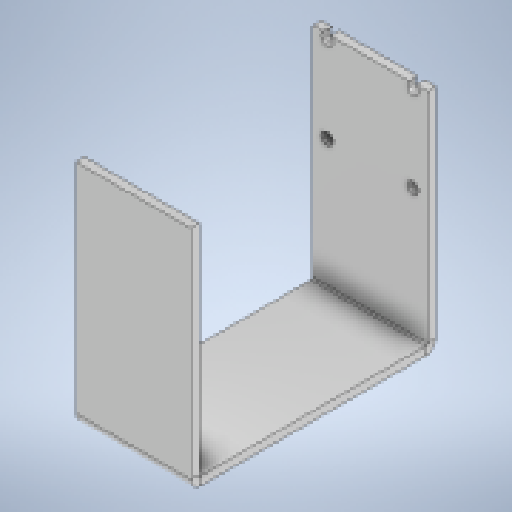
# Autodesk Inventor part: axis_25_top_frame
Saved by Autodesk Inventor 2025.2 (Build 292293000, 293)
## iProperties
Created: 2025-06-30
Part Number: axis_25_top_frame
Material: Aluminum 6061-AHC
Document SubType Name: Sheet Metal
Designer: LG
Density: 2.7 g/cm^3
Sheet Metal Rule: Default_mm
Appearance: Aluminum - Dark
Author: LG
Autodesk Inventor part; units mm, degrees
ref_plane "YZ Plane" through (0, 0, 0) normal (1, 0, 0) x (0, 1, 0)
ref_plane "XZ Plane" through (0, 0, 0) normal (0, 1, 0) x (-1, 0, 0)
ref_plane "XY Plane" through (0, 0, 0) normal (0, 0, 1) x (1, 0, 0)
sketch "Sketch1" plane through (0, 0, 0) normal (0, 1, 0) x (-1, 0, 0)
  line L0 (10.07, 20.05) -> (-10.07, 20.05)
  line L1 (-10.07, 20.05) -> (-10.07, -20.05)
  line L2 (-10.07, -20.05) -> (10.07, -20.05)
  line L3 (10.07, -20.05) -> (10.07, 20.05)
  point P0 (0, 0)
  dimension "d0" = 40.1
  dimension "d1" = 20.14
  dimension "d2" = 10.07
  dimension "d3" = 20.05
  measures "d0" distance of L2.end L0.start
  measures "d1" distance of L1.end L2.end
  measures "d2" distance from line of point (0, 0) L3
  measures "d3" distance from line of point (0, 0) L2
extrude "Plate1" add sketch "Sketch1" along normal blind 1.5
sketch "Sketch2" plane through (10.07, 0, 21.55) normal (0, 0, -1) x (-1, 0, 0)
  line L0 (20.14, 0) -> (0, 0)
  line L1 (0, 0) -> (0, 40.48)
  line L2 (0, 40.48) -> (20.14, 40.48)
  line L3 (20.14, 40.48) -> (20.14, 0)
  constraints: 8 end point
edge flange "Flange1" height 40.48 angle 90 thickness 1.5 bend radius 0.31 thickness toward (0, 0, -1) relief straight relief width 1.5 relief depth 0.75 corner gap 0.31 corner form 0 edges at (0, 1.5, 20.05) (0, 1.5, -20.05) wall of the first edge with corners at (-10.07, 0, 21.55) (10.07, 0, 21.55) (10.07, 40.48, 21.55) (-10.07, 40.48, 21.55)
bend "Bend1"
corner "Corner1"
sketch "Sketch3" plane through (10.07, 40.48, -21.55) normal (0, 0, -1) x (-1, 0, 0)
  circle A0 centre (17.595, -1.24) radius 0.7835 projected
  circle A1 centre (2.545, -1.24) radius 0.7835 projected
  circle A2 centre (2.545, -16.34) radius 0.7835 projected
  circle A3 centre (17.595, -16.34) radius 0.7835 projected
  point P0 (10.07, -40.48)
hole "Hole1" at (7.525, 39.24, -21.55) at (-7.525, 39.24, -21.55) at (-7.525, 24.14, -21.55) at (7.525, 24.14, -21.55) direction (0, 0, 1) diameter 2.1 depth 1.5
sketch "Sketch4" plane through (-10.07, 40.48, 21.55) normal (0, 0, 1) x (1, 0, 0)
  circle A0 centre (2.545, -1.24) radius 0.7835 projected
  circle A1 centre (17.595, -1.24) radius 0.7835 projected
  circle A2 centre (3.07, -8.86) radius 0.7835 projected
  circle A3 centre (17.07, -8.86) radius 0.7835 projected
  point P0 (10.07, -40.48)
sketch "Sketch5" plane through (-10.07, 40.48, 21.55) normal (0, 0, 1) x (1, 0, 0)
  circle A0 centre (10.07, -16.16) radius 0.7835 projected
  point P0 (10.07, -40.48)
hole "Hole2" at (-7.525, 39.24, 21.55) at (7.525, 39.24, 21.55) at (-7, 31.62, 21.55) at (7, 31.62, 21.55) direction (0, 0, -1) diameter 2.1 depth 1.5
hole "Hole3" at (0, 24.32, 21.55) direction (0, 0, -1) diameter 2.1 depth 1.5
equation "\"d20\" = Thickness"
equation "\"d27\" = Thickness"
equation "\"d34\" = Thickness"
equation "\"d4\" = Thickness"
equation "\"d5\" = BendReliefWidth"
equation "\"d6\" = BendReliefDepth"
equation "\"d7\" = MinimumRemnant"
equation "\"d8\" = TransitionRadius"
equation "\"d11\" = BendRadius"
equation "\"d12\" = CornerReliefSize"
equation "\"d13\" = GapSize"
equation "\"d14\" = JacobiRadiusSize"
equation "\"BendReliefWidth\" = Thickness"
equation "\"BendReliefDepth\" = 0.5 * Thickness"
equation "\"CornerReliefSize\" = 4 * Thickness"
equation "\"MinimumRemnant\" = 2 * Thickness"
equation "\"TransitionRadius\" = BendRadius"
equation "\"JacobiRadiusSize\" = BendRadius"
equation "\"GapSize\" = Thickness"
equation "\"Thickness\" = 1.5"
equation "\"BendRadius\" = 0.31"
body "Solid1"
